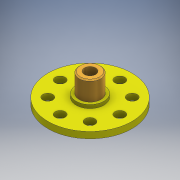
# Autodesk Inventor part: engraneGrande
Saved by Autodesk Inventor 2016 (Build 200138000, 138)
## iProperties
Created: 2016-09-20
Part Number: engraneGrande
Material: Plástico ABS
Document SubType Name: Modeling
Designer: i95sa
Density: 1.06 g/cm^3
Appearance: Suave - Blanco
Author: i95sa
Autodesk Inventor part; units mm, degrees
ref_plane "YZ Plane" through (0, 0, 0) normal (1, 0, 0) x (0, 1, 0)
ref_plane "XZ Plane" through (0, 0, 0) normal (0, 1, 0) x (-1, 0, 0)
ref_plane "XY Plane" through (0, 0, 0) normal (0, 0, 1) x (1, 0, 0)
sketch "Boceto1" plane through (0, 0, 0) normal (0, 0, 1) x (1, 0, 0)
  circle A0 centre (0, 0) radius 4.75
  circle A1 centre (0, 0) radius 2.5
  dimension "d0" = 9.5
  dimension "d1" = 5
  constraints: 2 centre point, 2 coincident
  measures "d0" diameter of A0
  measures "d1" diameter of A1
extrude "Extrusión1" add sketch "Boceto1" along normal blind 12.7
chamfer "Chaflán1" distance 1 angle 45 1 edges at (-4.75, 0, 0)
chamfer "Chaflán2" distance 0.5 angle 45 1 edges at (-4.75, 0, 12.7)
sketch "Boceto2" plane through (0, 0, 0) normal (0, 0, -1) x (-1, 0, 0)
  circle A0 centre (0, 0) radius 4.75
  circle A1 centre (0, 0) radius 6.075
  circle A2 centre (0, 0) radius 19.5
  circle A3 centre (0, 0) radius 4.25 projected
  circle A4 centre (0, 0) radius 18.4
  line L0 (0, 0) -> (0, -13.1)
  circle A5 centre (0, -13.1) radius 2.175
  circle A6 centre (9.2631, -9.2631) radius 2.175
  circle A7 centre (13.1, 0) radius 2.175
  circle A8 centre (9.2631, 9.2631) radius 2.175
  circle A9 centre (0, 13.1) radius 2.175
  circle A10 centre (-9.2631, 9.2631) radius 2.175
  circle A11 centre (-13.1, 0) radius 2.175
  circle A12 centre (-9.2631, -9.2631) radius 2.175
  dimension "d10" = 12.15
  dimension "d11" = 39
  dimension "d12" = 36.8
  dimension "d13" = 13.1
  dimension "d14" = 4.35
  dimension "d17" = 360
  constraints: 12 centre point, 7 coincident, 2 end point, 1 vertical, 23 other
  measures "d10" diameter of A1
  measures "d11" diameter of A2
  measures "d12" diameter of A4
  measures "d13" distance of L0.start L0.end
  measures "d14" diameter of A5
extrude "Extrusión2" add sketch "Boceto2" against normal blind 2.8 contours A1
extrude "Extrusión3" add sketch "Boceto2" against normal blind 2.8 contours A4
extrude "Extrusión4" add sketch "Boceto2" along normal blind 1.6 contours A1
extrude "Extrusión5" add sketch "Boceto2" against normal blind 4.3 contours A1
sketch "Boceto3" plane through (0, 0, 0) normal (0, 0, -1) x (-1, 0, 0)
  point P0 (0, 0)
